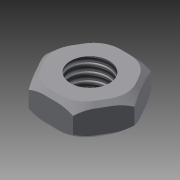
# Autodesk Inventor part: M2 Nut
Saved by Autodesk Inventor 2013 (Build 170138000, 138)
## iProperties
Created: 2012-10-31
Part Number: M2 Nut
Material: Generic
Document SubType Name: Modeling
Designer: uqgtayle
Density: 1 g/cm^3
Author: uqgtayle
Autodesk Inventor part; units mm, degrees
ref_plane "YZ Plane" through (0, 0, 0) normal (1, 0, 0) x (0, 1, 0)
ref_plane "XZ Plane" through (0, 0, 0) normal (0, 1, 0) x (-1, 0, 0)
ref_plane "XY Plane" through (0, 0, 0) normal (0, 0, 1) x (1, 0, 0)
sketch "Sketch1" plane through (0, 0, 0) normal (0, 0, 1) x (1, 0, 0)
  line L0 (1.1356, -2.0109) -> (-1.1737, -1.9889)
  line L1 (-1.1737, -1.9889) -> (-2.3093, 0.022)
  line L2 (-2.3093, 0.022) -> (-1.1356, 2.0109)
  line L3 (-1.1356, 2.0109) -> (1.1737, 1.9889)
  line L4 (1.1737, 1.9889) -> (2.3093, -0.022)
  line L5 (2.3093, -0.022) -> (1.1356, -2.0109)
  point P0 (0, 0)
  point P1 (0, 0)
  dimension "d0" = 4
  constraints: 12 end point, 1 coincident, 13 other
  measures "d0" distance between parallel lines of L0 L3
extrude "Extrusion1" add sketch "Sketch1" against normal blind 1.6
chamfer "Chamfer1" distance 0.2 angle 45 12 edges at (1.7415, 0.9834, 0) (0.0191, 1.9999, 0) (-1.7224, 1.0165, 0) (-1.7415, -0.9834, 0) (-0.0191, -1.9999, 0) (1.7224, -1.0165, 0) (1.7224, -1.0165, -1.6) (1.7415, 0.9834, -1.6) (0.0191, 1.9999, -1.6) (-1.7224, 1.0165, -1.6) (-1.7415, -0.9834, -1.6) (-0.0191, -1.9999, -1.6)
fillet "Fillet1" radius 2 12 edges at (-2.1938, 0.0209, -1.5) (-1.0788, 1.9104, -1.5) (1.115, 1.8895, -1.5) (2.1938, -0.0209, -1.5) (1.0788, -1.9104, -1.5) (-1.115, -1.8895, -1.5) (-1.115, -1.8895, -0.1) (-2.1938, 0.0209, -0.1) (-1.0788, 1.9104, -0.1) (1.115, 1.8895, -0.1) (2.1938, -0.0209, -0.1) (1.0788, -1.9104, -0.1)
sketch "Sketch2" plane through (0, 0, 0) normal (0, 0, 1) x (1, 0, 0)
  circle A0 centre (0, 0) radius 1
  dimension "d7" = 2
  constraints: 1 centre point, 1 coincident
  measures "d7" diameter of A0
extrude "Extrusion2" cut sketch "Sketch2" against normal through all
thread "Thread1" size "M2x0.4" class "6H" standard "ANSI Metric M Profile" full length
body "Solid1"
